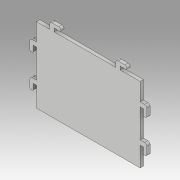
# Autodesk Inventor part: sides_instreamentboard
Saved by Autodesk Inventor 2019.3 (Build 233278000, 278)
## iProperties
Created: 2019-05-28
Part Number: sides_instreamentboard
Material: Generic
Document SubType Name: Modeling
Designer: Dave
Density: 1 g/cm^3
Appearance: Default
Author: Dave
Autodesk Inventor part; units mm, degrees
ref_plane "YZ Plane" through (0, 0, 0) normal (1, 0, 0) x (0, 1, 0)
ref_plane "XZ Plane" through (0, 0, 0) normal (0, 1, 0) x (-1, 0, 0)
ref_plane "XY Plane" through (0, 0, 0) normal (0, 0, 1) x (1, 0, 0)
sketch "Sketch1" plane through (0, 0, 0) normal (0, 0, 1) x (1, 0, 0)
  line L0 (0, 0) -> (94, 0)
  line L1 (94, 0) -> (94, 68)
  line L2 (94, 68) -> (0, 68)
  line L3 (0, 68) -> (0, 0)
  line L4 (12, 0) -> (20.5, 7)
  line L5 (20.5, 7) -> (73.5, 7)
  line L6 (73.5, 7) -> (82, 0)
  line L7 (0, 18) -> (-3, 18)
  line L8 (-3, 18) -> (-3, 13)
  line L9 (-4, 12) -> (-5, 12)
  line L10 (-6, 13) -> (-6, 20)
  line L11 (-4, 22) -> (0, 22)
  line L12 (0, 52) -> (-4, 52)
  line L13 (-6, 50) -> (-6, 43)
  line L14 (-5, 42) -> (-4, 42)
  line L15 (-3, 43) -> (-3, 48)
  line L16 (-3, 48) -> (0, 48)
  line L17 (94, 52) -> (98, 52)
  line L18 (100, 50) -> (100, 43)
  line L19 (99, 42) -> (98, 42)
  line L20 (97, 43) -> (97, 48)
  line L21 (97, 48) -> (94, 48)
  line L22 (94, 22) -> (98, 22)
  line L23 (100, 20) -> (100, 13)
  line L24 (99, 12) -> (98, 12)
  line L25 (97, 13) -> (97, 18)
  line L26 (97, 18) -> (94, 18)
  arc A0 (-4, 52) -> (-6, 50) centre (-4, 50) ccw
  arc A1 (-4, 22) -> (-6, 20) centre (-4, 20) ccw
  arc A2 (100, 20) -> (98, 22) centre (98, 20) ccw
  arc A3 (100, 50) -> (98, 52) centre (98, 50) ccw
  arc A4 (-6, 43) -> (-5, 42) centre (-5, 43) ccw
  arc A5 (-4, 42) -> (-3, 43) centre (-4, 43) ccw
  arc A6 (-6, 13) -> (-5, 12) centre (-5, 13) ccw
  arc A7 (-4, 12) -> (-3, 13) centre (-4, 13) ccw
  arc A8 (97, 43) -> (98, 42) centre (98, 43) ccw
  arc A9 (99, 42) -> (100, 43) centre (99, 43) ccw
  arc A10 (97, 13) -> (98, 12) centre (98, 13) ccw
  arc A11 (99, 12) -> (100, 13) centre (99, 13) ccw
  line L27 (12, 68) -> (12, 72)
  line L28 (14, 74) -> (20, 74)
  line L29 (22, 72) -> (22, 72)
  line L30 (21, 71) -> (16, 71)
  line L31 (16, 71) -> (16, 68)
  line L32 (72, 68) -> (72, 72)
  line L33 (74, 74) -> (80, 74)
  line L34 (82, 72) -> (82, 72)
  line L35 (81, 71) -> (76, 71)
  line L36 (76, 71) -> (76, 68)
  arc A12 (14, 74) -> (12, 72) centre (14, 72) ccw
  arc A13 (74, 74) -> (72, 72) centre (74, 72) ccw
  arc A14 (22, 72) -> (20, 74) centre (20, 72) ccw
  arc A15 (82, 72) -> (80, 74) centre (80, 72) ccw
  arc A16 (21, 71) -> (22, 72) centre (21, 72) ccw
  arc A17 (81, 71) -> (82, 72) centre (81, 72) ccw
  point P0 (-3, 12)
  point P1 (-6, 12)
  point P2 (-6, 22)
  point P3 (100, 52)
  point P4 (100, 22)
  point P5 (100, 12)
  point P6 (97, 12)
  point P7 (12, 74)
  point P8 (22, 74)
  point P9 (22, 71)
  point P10 (72, 74)
  point P11 (82, 74)
  point P12 (82, 71)
  dimension "d0" = 94
  dimension "d1" = 68
  dimension "d2" = 7
  dimension "d3" = 12
  dimension "d4" = 12
  dimension "d7" = 53
  dimension "d8" = 10
  dimension "d9" = 3
  dimension "d10" = 3
  dimension "d11" = 6
  dimension "d12" = 18
  dimension "d13" = 48
  dimension "d14" = 2
  dimension "d15" = 1
  dimension "d16" = 10
  dimension "d17" = 3
  dimension "d18" = 3
  dimension "d19" = 6
  dimension "d20" = 18
  dimension "d21" = 78
  dimension "d22" = 2
  dimension "d23" = 1
  constraints: 74 end point, 52 point on line, 36 point on circle, 36 tangent, 21 perpendicular, 18 centre point, 14 equal radius, 11 equal length, 4 parallel, 3 horizontal, 2 collinear, 1 vertical
  measures "d0" distance of L1.end L2.end
  measures "d1" distance of L0.end L1.end
  measures "d2" distance between parallel lines of L0 L5
  measures "d3" distance from line of L3 L4.start
  measures "d4" distance from line of L6.end L1
  measures "d7" distance of L4.end L5.end
  measures "d8" distance of point (-6, 12) point (-6, 22)
  measures "d9" distance of point (-3, 12) point (-6, 12)
  measures "d10" distance of L7.start L7.end
  measures "d11" distance of L7.end point (-3, 12)
  measures "d12" distance between parallel lines of L0 L7
  measures "d13" distance between parallel lines of L0 L16
  measures "d14" radius of A0
  measures "d15" radius of A4
  measures "d16" distance of point (12, 74) point (22, 74)
  measures "d17" distance of L30.end L31.end
  measures "d18" distance of point (22, 74) point (22, 71)
  measures "d19" distance of point (22, 71) L30.end
  measures "d20" distance between parallel lines of L1 L36
  measures "d21" distance between parallel lines of L1 L31
  measures "d22" radius of A12
  measures "d23" radius of A16
extrude "Extrusion1" add sketch "Sketch1" along normal blind 3
body "Solid1"
